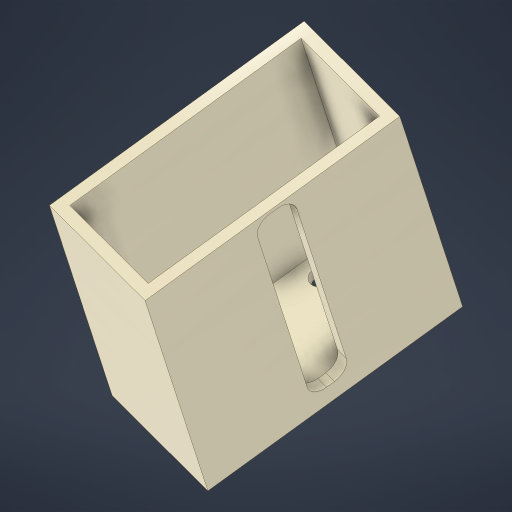
# Autodesk Inventor part: SLIDER
Saved by Autodesk Inventor 2023 (Build 270158000, 158)
## iProperties
Created: 2023-12-28
Part Number: SLIDER
Material: Steel, Alloy
Document SubType Name: Modeling
Designer: User
Density: 7.73 g/cm^3
Appearance: Light Beige
Author: User
Autodesk Inventor part; units mm, degrees
ref_plane "YZ Plane" through (0, 0, 0) normal (1, 0, 0) x (0, 1, 0)
ref_plane "XZ Plane" through (0, 0, 0) normal (0, 1, 0) x (-1, 0, 0)
ref_plane "XY Plane" through (0, 0, 0) normal (0, 0, 1) x (1, 0, 0)
sketch "Sketch1" plane through (0, 0, 0) normal (0, 0, 1) x (1, 0, 0)
  line L0 (-32.5, 16.5) -> (32.5, 16.5)
  line L1 (32.5, 16.5) -> (32.5, -16.5)
  line L2 (32.5, -16.5) -> (-32.5, -16.5)
  line L3 (-32.5, -16.5) -> (-32.5, 16.5)
  line L4 (-32.5, 16.5) -> (32.5, -16.5) construction
  line L5 (32.5, 16.5) -> (-32.5, -16.5) construction
  point P0 (0, 0)
  dimension "d0" = 65
  dimension "d1" = 33
  constraints: 12 end point, 2 midpoint, 2 parallel, 1 horizontal, 1 perpendicular
  measures "d0" distance of L1.end L2.end
  measures "d1" distance of L0.end L1.end
extrude "Extrusion1" add sketch "Sketch1" along normal blind 66
shell "Shell1" thickness 3 removed faces 1 at (-10.8333, 5.5, 66)
sketch "Sketch2" plane through (-32.5, -16.5, 0) normal (0, -1, 0) x (1, 0, 0)
  line L0 (33.5, 65) -> (31.5, 65)
  line L1 (27.5, 61) -> (27.5, 9)
  line L2 (31.5, 5) -> (33.5, 5)
  line L3 (37.5, 9) -> (37.5, 61)
  line L4 (32.5, 0) -> (32.5, 66) construction
  line L5 (65, 66) -> (0, 66) projected
  line L6 (0, 0) -> (65, 0) projected
  arc A0 (33.5, 5) -> (37.5, 9) centre (33.5, 9) ccw
  arc A1 (27.5, 9) -> (31.5, 5) centre (31.5, 9) ccw
  arc A2 (37.5, 61) -> (33.5, 65) centre (33.5, 61) ccw
  arc A3 (31.5, 65) -> (27.5, 61) centre (31.5, 61) ccw
  point P0 (37.5, 65)
  point P1 (27.5, 65)
  point P2 (27.5, 5)
  point P3 (37.5, 5)
  dimension "d5" = 10
  dimension "d6" = 60
  dimension "d7" = 5
  dimension "d10" = 4
  constraints: 10 end point, 8 point on circle, 8 point on line, 8 tangent, 4 centre point, 3 equal radius, 2 midpoint, 2 parallel, 1 horizontal, 1 perpendicular, 1 other
  measures "d5" distance of point (27.5, 5) point (37.5, 5)
  measures "d6" distance of point (27.5, 65) point (27.5, 5)
  measures "d7" distance from line of point (32.5, 0) L2
  measures "d10" radius of A0
extrude "Extrusion2" cut sketch "Sketch2" against normal up to surface (30 mm away)
sketch "Sketch3" plane through (0, 0, 0) normal (0, 0, -1) x (-1, 0, 0)
  line L0 (32.5, 16.5) -> (32.5, -16.5) projected
  line L1 (32.5, 0) -> (-32.5, 0) construction
  line L2 (-32.5, -16.5) -> (-32.5, 16.5) projected
  circle A0 centre (-15, -8) radius 2.5
  circle A1 centre (-15, 8) radius 2.5
  circle A2 centre (15, -8) radius 2.5
  circle A3 centre (15, 8) radius 2.5
  point P0 (0, 0)
  point P1 (0, 0)
  dimension "d11" = 5
  dimension "d12" = 5
  dimension "d13" = 5
  dimension "d14" = 5
  dimension "d15" = 8
  dimension "d16" = 8
  dimension "d17" = 30
  dimension "d18" = 15
  constraints: 4 centre point, 3 midpoint, 2 end point, 2 horizontal alignment, 2 vertical alignment
  measures "d11" diameter of A0
  measures "d12" diameter of A1
  measures "d13" diameter of A2
  measures "d14" diameter of A3
  measures "d15" distance from line of L1 A1.centre
  measures "d16" distance from line of L1 A0.centre
  measures "d17" distance of A2.centre A0.centre
  measures "d18" horizontal distance of A0.centre point (0, 0)
extrude "Extrusion3" cut sketch "Sketch3" against normal through all
body "Solid1"
